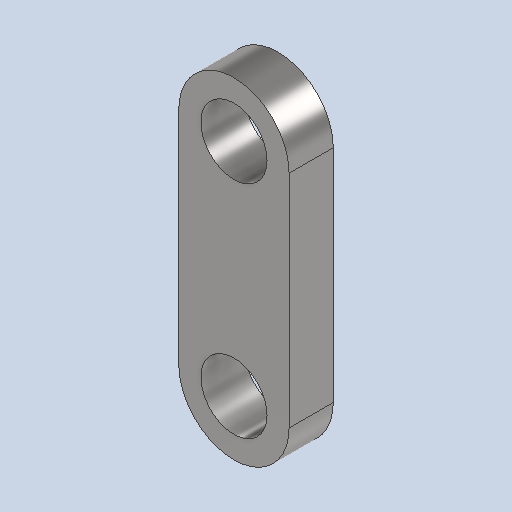
# Autodesk Inventor part: część L3
Saved by Autodesk Inventor 2022.1 (Build 261234020, 234B)
## iProperties
Created: 2022-05-02
Part Number: część L3
Material: Stal nierdzewna 440C
Document SubType Name: Modeling
Designer: Kacper Kaczmarski
Density: 7.75 g/cm^3
Appearance: Częściowo polerowany
Mass: 6.88173 g
Surface Area: 8.80442 cm^2
Volume: 0.887965 cm^3
Author: Kacper Kaczmarski
Autodesk Inventor part; units mm, degrees
ref_plane "YZ Plane" through (0, 0, 0) normal (1, 0, 0) x (0, 1, 0)
ref_plane "XZ Plane" through (0, 0, 0) normal (0, 1, 0) x (-1, 0, 0)
ref_plane "XY Plane" through (0, 0, 0) normal (0, 0, 1) x (1, 0, 0)
sketch "Szkic1" plane through (0, 0, 0) normal (0, 0, 1) x (1, 0, 0)
  line L0 (0, 0) -> (-10, 0)
  line L1 (-10, 0) -> (-10, 20)
  line L2 (-10, 20) -> (0, 20)
  line L3 (0, 20) -> (0, 0)
  arc A0 (0, 20) -> (-10, 20) centre (-5, 20) ccw
  arc A1 (-10, 0) -> (0, 0) centre (-5, 0) ccw
  circle A2 centre (-5, 20) radius 3
  circle A3 centre (-5, 0) radius 3
  dimension "d0" = 10
  dimension "d1" = 20
  dimension "d2" = 6
  dimension "d3" = 6
  constraints: 8 end point, 4 centre point, 4 point on circle, 4 tangent, 2 coincident, 2 parallel, 1 horizontal, 1 perpendicular
  measures "d0" distance of L1.end L2.end
  measures "d1" distance of L0.end L1.end
  measures "d2" diameter of A2
  measures "d3" diameter of A3
extrude "Wyciągnięcie proste1" add sketch "Szkic1" against normal blind 4 contours A1 L0 A3 | L0 A3 L1 L2 A2 L3 | L2 A2 A0
